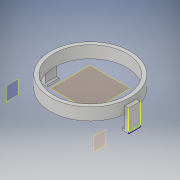
# Autodesk Inventor part: watchBodyOneTop
Saved by Autodesk Inventor 2019 (Build 230136000, 136)
## iProperties
Created: 2019-10-08
Part Number: watchBodyOneTop
Material: Generic
Document SubType Name: Modeling
Designer: Derek
Density: 1 g/cm^3
Appearance: Default
Author: Derek
Autodesk Inventor part; units mm, degrees
ref_plane "YZ Plane" through (0, 0, 0) normal (1, 0, 0) x (0, 1, 0)
ref_plane "XZ Plane" through (0, 0, 0) normal (0, 1, 0) x (-1, 0, 0)
ref_plane "XY Plane" through (0, 0, 0) normal (0, 0, 1) x (1, 0, 0)
ref_plane "Work Plane11" through (0, 7, 0) normal (0, 1, 0) x (1, 0, 0)
sketch "Sketch16" plane through (0, 7, 0) normal (0, 1, 0) x (1, 0, 0)
  circle A0 centre (0, 0) radius 22
  circle A1 centre (0, 0) radius 20 projected
  circle A2 centre (0, 0) radius 18.4
  dimension "d44" = 36.8
  constraints: 2 centre point, 2 coincident
  measures "d44" diameter of A2
extrude "Extrusion13" add sketch "Sketch16" along normal blind 6.7 contours A0
ref_plane "Work Plane3" through (24.0456, 0, 22.026) normal (1, 0, 0) x (0, 0, -1)
sketch "Sketch19" plane through (24.0456, 0, 22.026) normal (1, 0, 0) x (0, 0, -1)
  line L0 (19.05, 11.1125) -> (25.4, 11.1125)
  line L1 (25.4, 11.1125) -> (25.4, 7.9375)
  line L2 (25.4, 7.9375) -> (19.05, 7.9375)
  line L3 (19.05, 7.9375) -> (19.05, 11.1125)
  point P0 (22.026, 0)
  constraints: 8 end point, 2 parallel, 1 horizontal, 1 perpendicular
extrude "Extrusion15" add sketch "Sketch19" against normal blind 3
sketch "Sketch20" plane through (24.0456, 7.9375, -3.374) normal (0, -1, 0) x (1, 0, 0)
  line L0 (0, 6.35) -> (0, 0) projected
  line L1 (0, 6.35) -> (0, 0)
  line L2 (0, 0) -> (-2.3058, 0) projected
  line L3 (0, 0) -> (-2.3058, 0)
  arc A0 (-38.8494, -12.9001) -> (-38.8494, 19.6481) centre (-24.0456, 3.374) ccw projected
  arc A1 (-2.3058, 0) -> (-2.3058, 6.7481) centre (-24.0456, 3.374) ccw
  line L4 (0, 6.35) -> (-2.2478, 6.35) projected
  line L5 (0, 6.35) -> (-2.2478, 6.35)
  point P0 (-3, 0)
  point P1 (-3, 6.35)
  constraints: 6 end point, 3 point on circle, 2 collinear, 1 centre point, 1 perpendicular
extrude "Extrusion16" add sketch "Sketch20" along normal blind 9
sketch "Sketch21" plane through (24.0456, 0, 22.026) normal (1, 0, 0) x (0, 0, -1)
  line L0 (25.4, 0) -> (19.05, 0)
  line L1 (19.05, 11.1125) -> (19.05, -1.0625) projected
  line L2 (19.05, 0) -> (19.05, -1.0625)
  line L3 (25.4, 11.1125) -> (25.4, -1.0625) projected
  line L4 (19.05, -1.0625) -> (25.4, -1.0625)
  line L5 (25.4, -1.0625) -> (25.4, 0)
  point P0 (22.026, 0)
  constraints: 8 end point, 2 collinear, 1 perpendicular
ref_plane "Work Plane4" through (-24.0451, 0, 16.0514) normal (-1, 0, 0) x (0, 0, 1)
sketch "Sketch23" plane through (-24.0451, 0, 16.0514) normal (-1, 0, 0) x (0, 0, 1)
  line L0 (-19.4254, 11.1125) -> (-19.4254, 0) projected
  line L1 (-13.0754, 11.1125) -> (-13.0754, -1.0625) projected
  line L2 (-19.4254, 11.1125) -> (-13.0754, 11.1125)
  line L3 (-13.0754, 11.1125) -> (-13.0754, 7.9375)
  line L4 (-13.0754, 7.9375) -> (-19.4254, 7.9375)
  line L5 (-19.4254, 7.9375) -> (-19.4254, 11.1125)
  point P0 (-16.0514, 0)
  constraints: 8 end point, 2 parallel, 1 horizontal, 1 perpendicular, 1 point on line
extrude "Extrusion17" add sketch "Sketch23" against normal blind 3
sketch "Sketch24" plane through (-24.0451, 7.9375, -3.374) normal (0, -1, 0) x (1, 0, 0)
  arc A0 (2.2473, 6.35) -> (2.3053, 0) centre (24.0451, 3.374) ccw projected
  line L0 (2.3053, 0) -> (0, 0)
  line L1 (0, 0) -> (0, 6.35) projected
  line L2 (0, 0) -> (0, 6.35)
  line L3 (0, 6.35) -> (2.2473, 6.35) projected
  line L4 (0, 6.35) -> (2.2473, 6.35)
  arc A1 (2.2473, 6.35) -> (2.3053, 0) centre (24.0451, 3.374) ccw
  point P0 (3, 6.35)
  constraints: 6 end point, 2 point on circle, 1 centre point, 1 collinear, 1 concentric, 1 horizontal, 1 perpendicular
extrude "Extrusion18" add sketch "Sketch24" along normal blind 9
sketch "Sketch25" plane through (-24.0451, 0, 16.0514) normal (-1, 0, 0) x (0, 0, 1)
  line L0 (-19.4254, 11.1125) -> (-19.4254, -1.0625) projected
  line L1 (-13.0754, 0) -> (5.9486, 0) projected
  line L2 (-19.4254, -1.0625) -> (-13.0754, -1.0625)
  line L3 (-13.0754, -1.0625) -> (-13.0754, 0)
  line L4 (-13.0754, 0) -> (-19.4254, 0)
  line L5 (-19.4254, 0) -> (-19.4254, -1.0625)
  point P0 (-16.0514, 0)
  point P1 (0.2227, 0)
  constraints: 8 end point, 2 parallel, 1 horizontal, 1 perpendicular
extrude "Extrusion19" add sketch "Sketch25" against normal blind 3.5
sketch "Sketch26" plane through (24.0456, 0, 22.026) normal (1, 0, 0) x (0, 0, -1)
  line L0 (25.4, 11.1125) -> (25.4, 0) projected
  line L1 (19.05, -1.0625) -> (25.4, -1.0625) projected
  line L2 (25.4, 0) -> (19.05, 0)
  line L3 (19.05, 0) -> (19.05, -1.0625)
  line L4 (19.05, -1.0625) -> (25.4, -1.0625)
  line L5 (25.4, -1.0625) -> (25.4, 0)
  point P0 (22.026, 0)
  constraints: 8 end point, 2 parallel, 1 horizontal, 1 perpendicular
extrude "Extrusion20" add sketch "Sketch26" against normal blind 3.5
body "Solid1"
